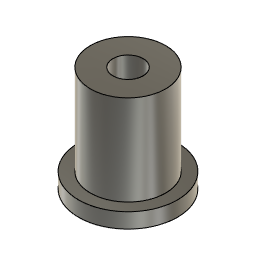
Vase (Autodesk Fusion 360 design; units mm, degrees)
Autodesk Fusion 360 part; units mm, degrees
sketch "Sketch1" plane through (0, 0, 0) normal (0, 0, 1) x (1, 0, 0)
  circle A0 centre (0, 0) radius 25
  circle A1 centre (0, 0) radius 32.8781
  dimension "d1" = 50
  dimension "d10" = 7.8781
  constraint coincident A0.centre A1.centre
  measures "d1" diameter of A0
extrude "Extrude2" add sketch "Sketch1" along normal blind 10 makes body 1
extrude "Extrude1" add sketch "Sketch1" along normal blind 70 separate body contours A0 makes body 2
hole "Hole2" at (0, 0, 70) direction (0, 0, -1) diameter 20 depth 55 tip angle 118 bodies 2
hole "Hole1" [suppressed]
named bodies: "Vase"
